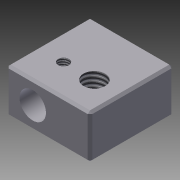
# Autodesk Inventor part: D-038
Saved by Autodesk Inventor 2015 (Build 190159000, 159)
## iProperties
Company: MARCHA TECHNOLOGY
Created: 2013-10-24
Part Number: D-038
Document SubType Name: Modeling
Designer: O.Martin
Density: 2.71 g/cm^3
Project: WITBOXprinter_K01
Description: HOT END DADO
Stock Number: 28656
Mass: 7.64059 g
Surface Area: 18.9694 cm^2
Volume: 2.81941 cm^3
Material: Aluminum-6061
Appearance: Aluminio mate
Author: O.Martin
Autodesk Inventor part; units mm, degrees
ref_plane "YZ Plane" through (0, 0, 0) normal (1, 0, 0) x (0, 1, 0)
ref_plane "XZ Plane" through (0, 0, 0) normal (0, 1, 0) x (-1, 0, 0)
ref_plane "XY Plane" through (0, 0, 0) normal (0, 0, 1) x (1, 0, 0)
sketch "Boceto1" plane through (0, 0, 0) normal (0, 0, 1) x (1, 0, 0)
  line L0 (9.5, -9.5) -> (-9.5, -9.5)
  line L1 (-9.5, -9.5) -> (-9.5, 9.5)
  line L2 (-9.5, 9.5) -> (9.5, 9.5)
  line L3 (9.5, 9.5) -> (9.5, -9.5)
  point P0 (0, 0)
  point P1 (0, -9.5)
  point P2 (-9.5, 0)
  dimension "d0" = 19
  dimension "d1" = 19
  constraints: 8 end point, 2 midpoint, 2 parallel, 1 horizontal, 1 horizontal alignment, 1 perpendicular, 1 vertical alignment
  measures "d0" distance of L0.start L0.end
  measures "d1" distance of L0.end L1.end
extrude "Extrusión1" add sketch "Boceto1" along normal mid plane 10
sketch "Boceto2" plane through (0, 0, 5) normal (0, 0, 1) x (1, 0, 0)
  line L0 (9.5, -9.5) -> (-9.5, -9.5) projected
  line L1 (-9.5, 9.5) -> (9.5, 9.5) projected
  line L2 (0, -9.5) -> (0, 9.5) construction
  point P0 (3.5, -2.5)
  dimension "d4" = 3.5
  dimension "d40" = 12
  constraints: 2 end point, 2 midpoint
  measures "d4" distance from line of L2 point (3.5, -2.5)
  measures "d40" distance from line of L1 point (3.5, -2.5)
hole "Agujero1" at (3.5, -2.5, 5) direction (0, 0, -1) diameter 4.917 end through all thread size "M6x1" class "6H" standard "ISO Metric profile"
sketch "Boceto3" plane through (-9.5, 9.5, 5) normal (0, 1, 0) x (1, 0, 0)
  line L0 (0, 0) -> (19, 0) projected
  line L1 (19, 10) -> (0, 10) projected
  line L2 (9.5, 0) -> (9.5, 10) construction
  line L3 (10.5415, 10) -> (15.4585, 10) projected
  point P0 (6, 5)
  point P1 (9.5, 5)
  point P2 (13, 5)
  point P3 (13, 10)
  dimension "d12" = 3.5
  constraints: 4 midpoint, 2 end point, 2 horizontal alignment, 1 vertical alignment
  measures "d12" distance from line of L2 point (6, 5)
hole "Agujero2" at (-3.5, 9.5, 0) direction (0, -1, 0) diameter 6 end through all
hole "Agujero3" at (3.5, 9.5, 0) direction (0, -1, 0) diameter 2.459 depth 7 tip angle 118 thread size "M3x0.5" class "6H" standard "ISO Metric profile"
sketch "Boceto4" plane through (0, 0, 5) normal (0, 0, 1) x (1, 0, 0)
  line L0 (-9.5, 9.5) -> (9.5, 9.5)
  line L1 (-6.5, 9.5) -> (-0.5, 9.5) projected
  circle A0 centre (3.5, -2.5) radius 2.4585 projected
  point P0 (-3.5, -2.5)
  point P1 (-3.5, 9.5)
  constraints: 2 end point, 1 horizontal alignment, 1 midpoint, 1 vertical alignment
hole "Agujero4" at (-3.5, -2.5, 5) direction (0, 0, -1) diameter 2.459 depth 6 tip angle 118 thread size "M3x0.5" class "6H" standard "ISO Metric profile"
chamfer "Chaflán1" distance 0.5 angle 45 12 edges at (0, 9.5, 5) (9.5, 0, 5) (0, -9.5, 5) (-9.5, 0, 5) (9.5, 9.5, 0) (0, 9.5, -5) (9.5, 0, -5) (9.5, -9.5, 0) (-9.5, 9.5, 0) (-9.5, 0, -5) (0, -9.5, -5) (-9.5, -9.5, 0)
body "Solid1"
